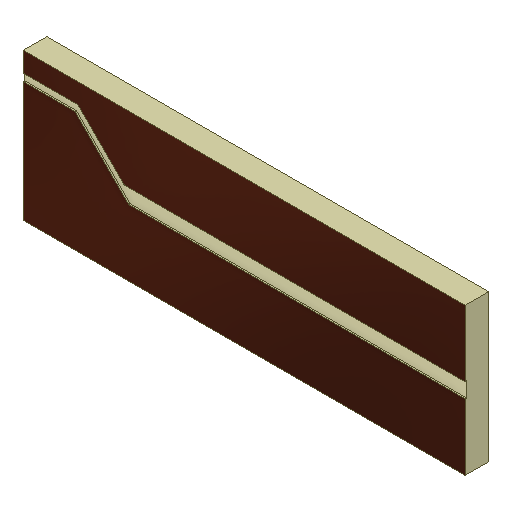
# Autodesk Inventor part: CNCM_FR4_Measurement_Rail_Contacts
Saved by Autodesk Inventor 2026.1 (Build 301233000, 233)
## iProperties
Created: 2018-07-19
Part Number: CNCM_FR4_Measurement_Rail_Contacts
Material: Polypropylene
Document SubType Name: Modeling
Designer: Andrzej
Density: 0.899 g/cm^3
Appearance: Smooth - Ash
Author: Andrzej
Autodesk Inventor part; units mm, degrees
ref_plane "YZ Plane" through (0, 0, 0) normal (1, 0, 0) x (0, 1, 0)
ref_plane "XZ Plane" through (0, 0, 0) normal (0, 1, 0) x (-1, 0, 0)
ref_plane "XY Plane" through (0, 0, 0) normal (0, 0, 1) x (1, 0, 0)
sketch "Sketch1" plane through (0, 0, 0) normal (0, 0, 1) x (1, 0, 0)
  line L0 (-15, 5) -> (15, 5)
  line L1 (15, 5) -> (15, -5)
  line L2 (15, -5) -> (-15, -5)
  line L3 (-15, -5) -> (-15, 5)
  point P0 (0, 0)
  dimension "d0" = 30
  dimension "d1" = 10
  dimension "d10" = 5
  dimension "d11" = 15
  constraints: 8 end point, 2 parallel, 1 horizontal, 1 perpendicular
  measures "d0" distance of L1.end L2.end
  measures "d1" distance of L0.end L1.end
  measures "d10" distance from line of L0 point (0, 0)
  measures "d11" distance from line of L3 point (0, 0)
extrude "Extrusion1" add sketch "Sketch1" along normal blind 1.5
sketch "Sketch2" plane through (0, 0, 1.5) normal (0, 0, 1) x (1, 0, 0)
  line L0 (15, 5) -> (-15, 5) projected
  line L1 (-15, 5) -> (-15, -5) projected
  line L2 (-15, -5) -> (15, -5) projected
  line L3 (15, -5) -> (15, 5) projected
  line L4 (-15, 5) -> (-15, -5) projected
  line L5 (-15, 3.65) -> (-11.2929, 3.65)
  line L6 (-15, 3.15) -> (-11.5, 3.15)
  line L7 (-11.5, 3.15) -> (-7.85, -0.5)
  line L8 (-11.5, 3.15) -> (-4.55, 3.15) construction
  line L9 (15, -5) -> (15, 5) projected
  line L10 (-7.85, -0.5) -> (15, -0.5)
  line L11 (-8.1429, 0.5) -> (15, 0.5)
  line L12 (-11.2929, 3.65) -> (-8.1429, 0.5)
  point P0 (0, 0)
  point P1 (-15, 3.4)
  dimension "d4" = 1.6
  dimension "d5" = 0.25
  dimension "d6" = 0.25
  dimension "d8" = 10
  dimension "d13" = 45
  dimension "d14" = 3.5
  dimension "d17" = 0.5
  constraints: 14 end point, 5 point on line, 2 horizontal, 2 parallel, 2 perpendicular
  measures "d4" distance from line of L0 point (-15, 3.4)
  measures "d5" distance from line of point (-15, 3.4) L5
  measures "d6" distance from line of point (-15, 3.4) L6
  measures "d8" distance between parallel lines of L2 L0
  measures "d13" angle of L7 L8
  measures "d14" distance of L6.start L6.end
  measures "d17" distance from line of L10 point (0, 0)
extrude "Extrusion2" add sketch "Sketch2" along normal blind 0.1 contours L3 L11 L12 L5 L1 L0 | L3 L2 L1 L6 L7 L10
equation "\"d10\" = 0.5 * d1"
equation "\"d11\" = 0.5 * d0"
equation "\"d6\" = d5"
equation "\"d17\" = d16"
equation "\"d16\" = 0.5"
body "Solid1"
